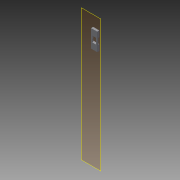
# Autodesk Inventor part: boardHolderv2
Saved by Autodesk Inventor 2014 (Build 180170000, 170)
## iProperties
Created: 2014-01-11
Part Number: boardHolderv2
Material: Generic
Document SubType Name: Modeling
Designer: intern
Density: 1 g/cm^3
Appearance: Default
Author: intern
Autodesk Inventor part; units mm, degrees
ref_plane "YZ Plane" through (0, 0, 0) normal (1, 0, 0) x (0, 1, 0)
ref_plane "XZ Plane" through (0, 0, 0) normal (0, 1, 0) x (-1, 0, 0)
ref_plane "XY Plane" through (0, 0, 0) normal (0, 0, 1) x (1, 0, 0)
ref_plane "Work Plane1" through (0, 0, 0) normal (0, 0, 1) x (1, 0, 0)
sketch "Sketch1" plane through (0, 0, 0) normal (0, 0, 1) x (1, 0, 0)
  circle A0 centre (26.9875, 590.55) radius 15.621 projected
  line L0 (11.3665, 606.171) -> (42.6085, 606.171)
  line L1 (42.6085, 606.171) -> (42.6085, 574.929)
  line L2 (42.6085, 574.929) -> (11.3665, 574.929)
  line L3 (11.3665, 574.929) -> (11.3665, 606.171)
  line L4 (11.3665, 606.171) -> (42.6085, 574.929) construction
  line L5 (42.6085, 606.171) -> (11.3665, 574.929) construction
  line L6 (10.8585, 637.921) -> (43.1165, 637.921)
  line L7 (43.1165, 637.921) -> (43.1165, 543.179)
  line L8 (43.1165, 543.179) -> (10.8585, 543.179)
  line L9 (10.8585, 543.179) -> (10.8585, 637.921)
  line L10 (10.8585, 637.921) -> (43.1165, 543.179) construction
  line L11 (43.1165, 637.921) -> (10.8585, 543.179) construction
  line L12 (42.6085, 606.171) -> (43.1165, 606.171)
  line L13 (11.3665, 606.171) -> (10.8585, 606.171)
  line L14 (11.3665, 574.929) -> (10.8585, 574.929)
  line L15 (42.6085, 574.929) -> (43.1165, 574.929)
  point P0 (0, 0)
  dimension "d0" = 32.258
  dimension "d1" = 94.742
  constraints: 32 end point, 5 equal length, 5 perpendicular, 4 midpoint, 4 point on line, 3 horizontal, 1 vertical
  measures "d0" distance of L7.end L8.end
  measures "d1" distance of L6.end L7.end
extrude "Extrusion1" add sketch "Sketch1" along normal blind 5.08 contours L0 L13 L9 L6 L7 L12 | L2 L15 L7 L8 L9 L14
sketch "Sketch2" plane through (0, 0, 5.08) normal (0, 0, 1) x (1, 0, 0)
  line L0 (10.8585, 606.171) -> (43.1165, 606.171) projected
  line L1 (43.1165, 606.171) -> (43.1165, 637.921) projected
  line L2 (43.1165, 637.921) -> (10.8585, 637.921) projected
  circle A0 centre (26.9875, 590.55) radius 8.9481 projected
  line L3 (35.8299, 591.9213) -> (35.0382, 597.0264) projected
  line L4 (35.0382, 597.0264) -> (30.2211, 598.8934) projected
  line L5 (36.6216, 586.8161) -> (35.8299, 591.9213) projected
  line L6 (32.5963, 583.5779) -> (36.6216, 586.8161) projected
  line L7 (28.5709, 580.3397) -> (32.5963, 583.5779) projected
  line L8 (23.7539, 582.2066) -> (28.5709, 580.3397) projected
  line L9 (28.1112, 583.3043) -> (33.8243, 587.9003) projected
  line L10 (33.8243, 587.9003) -> (32.7007, 595.146) projected
  line L11 (32.7007, 595.146) -> (25.8638, 597.7957) projected
  line L12 (25.8638, 597.7957) -> (20.1507, 593.1997) projected
  line L13 (20.1507, 593.1997) -> (21.2743, 585.954) projected
  line L14 (21.2743, 585.954) -> (28.1112, 583.3043) projected
  line L15 (28.5709, 580.3397) -> (18.9368, 584.0736) projected
  line L16 (18.9368, 584.0736) -> (17.3534, 594.2839) projected
  line L17 (17.3534, 594.2839) -> (25.4041, 600.7603) projected
  line L18 (25.4041, 600.7603) -> (35.0382, 597.0264) projected
  line L19 (35.0382, 597.0264) -> (36.6216, 586.8161) projected
  line L20 (36.6216, 586.8161) -> (28.5709, 580.3397) projected
  line L21 (43.1165, 574.929) -> (10.8585, 574.929) projected
  line L22 (10.8585, 574.929) -> (10.8585, 543.179) projected
  line L23 (10.8585, 543.179) -> (43.1165, 543.179) projected
  line L24 (43.1165, 543.179) -> (43.1165, 574.929) projected
  line L25 (43.1165, 637.921) -> (37.3198, 637.921)
  line L26 (37.3198, 543.179) -> (43.1165, 543.179)
  line L27 (43.1165, 543.179) -> (43.1165, 637.921)
  line L28 (10.8585, 543.179) -> (16.6552, 543.179)
  line L29 (16.6552, 637.921) -> (10.8585, 637.921)
  line L30 (10.8585, 637.921) -> (10.8585, 543.179)
  line L31 (37.3198, 637.921) -> (16.6552, 637.921)
  line L32 (16.6552, 637.921) -> (16.6552, 606.171)
  line L33 (16.6552, 606.171) -> (37.3198, 606.171)
  line L34 (37.3198, 606.171) -> (37.3198, 637.921)
  line L35 (37.3198, 574.929) -> (16.6552, 574.929)
  line L36 (16.6552, 574.929) -> (16.6552, 543.179)
  line L37 (16.6552, 543.179) -> (37.3198, 543.179)
  line L38 (37.3198, 543.179) -> (37.3198, 574.929)
  circle A1 centre (26.9875, 590.55) radius 10.9728
  line L39 (37.3198, 606.171) -> (37.3198, 594.2439)
  line L40 (37.3198, 586.8561) -> (37.3198, 574.929)
  line L41 (43.1165, 637.921) -> (43.1165, 543.179)
  line L42 (43.1165, 543.179) -> (37.3198, 543.179)
  line L43 (37.3198, 637.921) -> (43.1165, 637.921)
  line L44 (16.6552, 637.921) -> (16.6552, 594.2439)
  line L45 (16.6552, 586.8561) -> (16.6552, 543.179)
  line L46 (10.8585, 543.179) -> (43.1165, 543.179)
  line L47 (43.1165, 543.179) -> (43.1165, 574.929)
  line L48 (43.1165, 574.929) -> (10.8585, 574.929)
  line L49 (10.8585, 574.929) -> (10.8585, 543.179)
  line L50 (10.8585, 637.921) -> (43.1165, 637.921)
  line L51 (43.1165, 637.921) -> (43.1165, 606.171)
  line L52 (43.1165, 606.171) -> (10.8585, 606.171)
  line L53 (10.8585, 606.171) -> (10.8585, 637.921)
  line L54 (16.6552, 574.929) -> (10.8585, 574.929)
  line L55 (10.8585, 574.929) -> (10.8585, 543.179)
  line L56 (10.8585, 543.179) -> (16.6552, 543.179)
  line L57 (16.6552, 543.179) -> (16.6552, 574.929)
  line L58 (43.1165, 574.929) -> (37.3198, 574.929)
  line L59 (37.3198, 574.929) -> (37.3198, 543.179)
  line L60 (37.3198, 543.179) -> (43.1165, 543.179)
  line L61 (43.1165, 543.179) -> (43.1165, 574.929)
  line L62 (16.6552, 586.8561) -> (16.6552, 574.929)
  line L63 (16.6552, 574.929) -> (10.8585, 574.929)
  line L64 (10.8585, 574.929) -> (10.8585, 606.171)
  line L65 (10.8585, 606.171) -> (16.6552, 606.171)
  line L66 (16.6552, 606.171) -> (16.6552, 594.2439)
  line L67 (37.3198, 574.929) -> (37.3198, 586.8561)
  line L68 (37.3198, 594.2439) -> (37.3198, 606.171)
  line L69 (43.1165, 606.171) -> (37.3198, 606.171)
  line L70 (43.1165, 606.171) -> (43.1165, 574.929)
  line L71 (43.1165, 574.929) -> (37.3198, 574.929)
  line L72 (43.1165, 574.929) -> (10.8585, 574.929)
  point P0 (0, 0)
  dimension "d4" = 21.9456
  constraints: 96 end point, 16 parallel, 14 perpendicular, 8 collinear, 8 horizontal, 4 point on circle, 4 point on line, 4 vertical, 1 centre point
  measures "d4" diameter of A1
extrude "Extrusion3" add sketch "Sketch2" along normal blind 6.0706 contours L30 L2 L32 L0 | L0 L44 A1 L45 L21 L30 | L32 L2 L34 L0 | L21 L36 L23 L22 | L34 L2 L1 L0 | L0 L27 L21 L40 A1 L39 | L21 L38 L23 L36 | L21 L24 L23 L38
body "Solid1"
